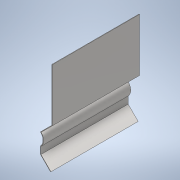
# Autodesk Inventor part: front
Saved by Autodesk Inventor 2020 (Build 240168000, 168)
## iProperties
Created: 2020-04-30
Part Number: front
Material: Generic
Document SubType Name: Modeling
Designer: LENOVO
Density: 1 g/cm^3
Appearance: Default
Author: LENOVO
Autodesk Inventor part; units mm, degrees
ref_plane "YZ Plane" through (0, 0, 0) normal (1, 0, 0) x (0, 1, 0)
ref_plane "XZ Plane" through (0, 0, 0) normal (0, 1, 0) x (-1, 0, 0)
ref_plane "XY Plane" through (0, 0, 0) normal (0, 0, 1) x (1, 0, 0)
sketch "Sketch2" plane through (0, 0, 0) normal (0, 0, 1) x (1, 0, 0)
  line L0 (100, 150) -> (100, -150)
  line L1 (100, -150) -> (36.4382, -213.5618)
  line L2 (35.3571, -283.1536) -> (35.3571, -323.1554)
  line L3 (35.3571, -323.1554) -> (91.9257, -379.7239)
  arc A0 (35.3571, -283.1536) -> (36.4382, -213.5618) centre (0, -247.8) ccw
  line L4 (97, -148.7574) -> (32.197, -213.5604)
  line L5 (97, -148.7574) -> (97, 144.1913)
  line L6 (87.683, -379.7239) -> (32.3571, -324.398)
  line L7 (91.9257, -379.7239) -> (87.683, -379.7239)
  arc A1 (32.3571, -281.8884) -> (32.197, -213.5604) centre (0, -247.8) ccw
  line L8 (32.3571, -281.8884) -> (32.3571, -324.398)
  line L9 (100, 150) -> (97, 150)
  line L10 (97, 144.031) -> (97, 150)
  point P0 (97, 144.0372)
  dimension "d26" = 3
  dimension "d28" = 3
  dimension "d29" = 94
  dimension "d30" = 3
  dimension "d31" = 3
  dimension "d32" = 3
  dimension "d33" = 3
  constraints: 22 end point, 4 point on circle, 3 parallel, 2 centre point, 2 horizontal, 2 vertical, 1 coincident, 1 point on line
  measures "d26" distance between parallel lines of L3 L6
  measures "d28" distance between parallel lines of L4 L1
  measures "d29" diameter of A1
  measures "d30" radial gap between concentric circles of A1 A0
  measures "d31" distance between parallel lines of L8 L2
  measures "d32" distance between parallel lines of L5 L0
  measures "d33" distance of L0.start L9.end
extrude "Extrusion2" add sketch "Sketch2" against normal blind 494
body "Solid2"
